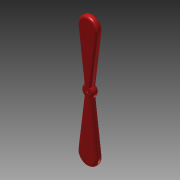
# Autodesk Inventor part: Prop
Saved by Autodesk Inventor 2013 (Build 170138000, 138)
## iProperties
Created: 2013-06-27
Part Number: Prop
Material: Nylon 6/6
Document SubType Name: Modeling
Designer: Kyle
Density: 1 g/cm^3
Author: Kyle
Autodesk Inventor part; units mm, degrees
ref_plane "YZ Plane" through (0, 0, 0) normal (1, 0, 0) x (0, 1, 0)
ref_plane "XZ Plane" through (0, 0, 0) normal (0, 1, 0) x (-1, 0, 0)
ref_plane "XY Plane" through (0, 0, 0) normal (0, 0, 1) x (1, 0, 0)
sketch "Sketch1" plane through (0, 0, 0) normal (0, 0, 1) x (1, 0, 0)
  circle A0 centre (0, 0) radius 0.635
  line L0 (-1.905, 2.54) -> (-5.08, 27.94)
  line L1 (5.08, 27.94) -> (1.905, 2.54)
  line L2 (-5.08, -27.94) -> (-1.905, -2.54)
  line L3 (1.905, -2.54) -> (5.08, -27.94)
  arc A1 (-5.08, -27.94) -> (5.08, -27.94) centre (0, -28.575) ccw
  arc A2 (5.08, 27.94) -> (-5.08, 27.94) centre (0, 28.575) ccw
  arc A3 (-1.905, 2.54) -> (-1.905, -2.54) centre (0, 0) ccw
  arc A4 (1.905, -2.54) -> (1.905, 2.54) centre (0, 0) ccw
  dimension "d0" = 1.27
  dimension "d3" = 2.54
  dimension "d4" = 1.905
  dimension "d5" = 2.54
  dimension "d6" = 1.905
  dimension "d7" = 25.4
  dimension "d8" = 25.4
  dimension "d9" = 3.175
  dimension "d10" = 3.175
  dimension "d11" = 25.4
  dimension "d12" = 25.4
  dimension "d13" = 3.175
  dimension "d14" = 3.175
  constraints: 8 end point, 8 point on circle, 5 centre point, 3 tangent, 1 coincident
  measures "d0" diameter of A0
  measures "d3" vertical distance of L0.start point (0, 0)
  measures "d4" horizontal distance of L0.start point (0, 0)
  measures "d5" vertical distance of L1.end point (0, 0)
  measures "d6" horizontal distance of L1.end point (0, 0)
  measures "d7" vertical distance of L2.end L2.start
  measures "d8" vertical distance of L3.start L3.end
  measures "d9" horizontal distance of L3.end L3.start
  measures "d10" horizontal distance of L2.end L2.start
  measures "d11" vertical distance of L1.end L1.start
  measures "d12" vertical distance of L0.start L0.end
  measures "d13" horizontal distance of L0.end L0.start
  measures "d14" horizontal distance of L1.end L1.start
extrude "Extrusion1" add sketch "Sketch1" along normal blind 3.175
fillet "Fillet1" radius 1.27 16 edges at (0, 33.6945, 3.175) (-3.4925, 15.24, 3.175) (3.4925, 15.24, 3.175) (0, -33.6945, 3.175) (-3.4925, -15.24, 3.175) (3.4925, -15.24, 3.175) (0, -33.6945, 0) (-3.4925, -15.24, 0) (3.4925, -15.24, 0) (0, 33.6945, 0) (-3.4925, 15.24, 0) (3.4925, 15.24, 0) (3.175, 0, 3.175) (-3.175, 0, 3.175) (3.175, 0, 0) (-3.175, 0, 0)
body "Solid1"
